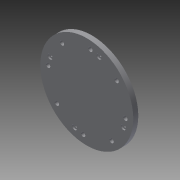
# Autodesk Inventor part: bay container 10 bottom
Saved by Autodesk Inventor 2015 (Build 190159000, 159)
## iProperties
Created: 2014-10-01
Part Number: bay container 10 bottom
Material: Generic
Document SubType Name: Modeling
Designer: ericd_000
Density: 1 g/cm^3
Appearance: Default
Author: ericd_000
Autodesk Inventor part; units mm, degrees
ref_plane "YZ Plane" through (0, 0, 0) normal (1, 0, 0) x (0, 1, 0)
ref_plane "XZ Plane" through (0, 0, 0) normal (0, 1, 0) x (-1, 0, 0)
ref_plane "XY Plane" through (0, 0, 0) normal (0, 0, 1) x (1, 0, 0)
sketch "Sketch1" plane through (0, 0, 0) normal (0, 1, 0) x (-1, 0, 0)
  circle A0 centre (0, 0) radius 65
  dimension "d0" = 130
  constraints: 1 centre point, 1 coincident
  measures "d0" diameter of A0
extrude "Extrusion1" add sketch "Sketch1" along normal blind 7
sketch "Sketch2" plane through (0, 7, 0) normal (0, 1, 0) x (1, 0, 0)
  circle A0 centre (-54, -5.0532) radius 3
  circle A1 centre (-34.6106, -41.7569) radius 3
  circle A2 centre (5.0532, -54) radius 3
  circle A3 centre (41.7569, -34.6106) radius 3
  circle A4 centre (54, 5.0532) radius 3
  circle A5 centre (34.6106, 41.7569) radius 3
  circle A6 centre (-5.0532, 54) radius 3
  circle A7 centre (-41.7569, 34.6106) radius 3
  point P0 (0, 0)
  dimension "d3" = 6
  dimension "d4" = 54
  dimension "d7" = 360
  constraints: 8 centre point, 17 other
  measures "d3" diameter of A0
  measures "d4" horizontal distance of point (0, 0) A0.centre
extrude "Extrusion2" cut sketch "Sketch2" against normal through all
sketch "Sketch3" plane through (0, 7, 0) normal (0, 1, 0) x (1, 0, 0)
  circle A0 centre (-51.2366, -17.0532) radius 1.5
  circle A1 centre (-54, -5.0532) radius 3 projected
  circle A2 centre (17.0532, -51.2366) radius 1.5
  circle A3 centre (51.2366, 17.0532) radius 1.5
  circle A4 centre (-17.0532, 51.2366) radius 1.5
  circle A5 centre (-34.6106, -41.7569) radius 3 projected
  point P0 (0, 0)
  dimension "d13" = 3
  dimension "d16" = 360
  dimension "d31" = 12
  dimension "d33" = 54
  constraints: 4 centre point, 9 other
  measures "d13" diameter of A0
  measures "d31" vertical distance of A1.centre A0.centre
  measures "d33" distance of point (0, 0) A0.centre
extrude "Extrusion3" cut sketch "Sketch3" against normal through all contours A0 | A2 | A3 | A4
sketch "Sketch4" plane through (0, 0, 0) normal (0, -1, 0) x (1, 0, 0)
  circle A0 centre (17.0532, 51.2366) radius 3.5
  circle A1 centre (17.0532, 51.2366) radius 1.5 projected
  circle A2 centre (-51.2366, 17.0532) radius 3.5
  circle A3 centre (-17.0532, -51.2366) radius 3.5
  circle A4 centre (51.2366, -17.0532) radius 3.5
  point P0 (0, 0)
  dimension "d20" = 7
  dimension "d23" = 360
  constraints: 4 centre point, 1 concentric, 9 other
  measures "d20" diameter of A0
extrude "Extrusion4" cut sketch "Sketch4" against normal blind 2
sketch "Sketch5" plane through (0, 7, 0) normal (0, 1, 0) x (1, 0, 0)
  circle A0 centre (0, 0) radius 6
  dimension "d27" = 12
  constraints: 1 centre point, 1 coincident
  measures "d27" diameter of A0
extrude "Extrusion5" add sketch "Sketch5" along normal blind 2
body "Solid1"
